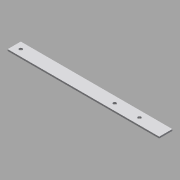
# Autodesk Inventor part: Long Arm
Saved by Autodesk Inventor 2013 (Build 170138000, 138)
## iProperties
Created: 2013-02-08
Part Number: Long Arm
Material: Aluminum 6061-AHC
Document SubType Name: Modeling
Designer: Naphat
Density: 1 g/cm^3
Author: Naphat
Autodesk Inventor part; units mm, degrees
ref_plane "YZ Plane" through (0, 0, 0) normal (1, 0, 0) x (0, 1, 0)
ref_plane "XZ Plane" through (0, 0, 0) normal (0, 1, 0) x (-1, 0, 0)
ref_plane "XY Plane" through (0, 0, 0) normal (0, 0, 1) x (1, 0, 0)
sketch "Sketch1" plane through (0, 0, 0) normal (0, 1, 0) x (-1, 0, 0)
  line L0 (0, 0) -> (0, 25.4)
  line L1 (0, 25.4) -> (254, 25.4)
  line L2 (254, 25.4) -> (254, 0)
  line L3 (254, 0) -> (0, 0)
  dimension "d0" = 25.4
  dimension "d1" = 254
  constraints: 8 end point, 2 perpendicular, 1 parallel, 1 vertical
  measures "d0" distance of L0.start L0.end
  measures "d1" distance of L0.end L1.end
extrude "Extrusion1" add sketch "Sketch1" along normal blind 3
sketch "Sketch2" plane through (0, 3, 0) normal (0, 1, 0) x (1, 0, 0)
  line L0 (0, -25.4) -> (0, 0) projected
  line L1 (0, 0) -> (-254, 0) projected
  line L2 (-254, 0) -> (-254, -25.4) projected
  line L3 (-254, -25.4) -> (0, -25.4) projected
  line L4 (-254, 0) -> (-254, -12.7) construction
  line L5 (-254, 0) -> (-241.3, 0) construction
  line L6 (0, 0) -> (-12.7, 0) construction
  line L7 (0, 0) -> (0, -12.7) construction
  line L8 (0, -12.7) -> (-254, -12.7) construction
  line L9 (-241.3, 0) -> (-241.3, -25.4) construction
  line L10 (-12.7, 0) -> (-12.7, -25.4) construction
  circle A0 centre (-241.3, -12.7) radius 3.175
  circle A1 centre (-12.7, -12.7) radius 3.175
  dimension "d4" = 12.7
  dimension "d5" = 12.7
  dimension "d6" = 12.7
  dimension "d7" = 12.7
  dimension "d8" = 6.35
  dimension "d9" = 6.35
  constraints: 14 end point, 4 midpoint, 4 point on line, 2 centre point, 2 perpendicular
  measures "d4" distance of L1.end L4.end
  measures "d5" distance of L1.end L5.end
  measures "d6" distance of L0.end L6.end
  measures "d7" distance of L0.end L7.end
  measures "d8" diameter of A0
  measures "d9" diameter of A1
hole "Hole1" at (-12.7, 3, 12.7) at (-241.3, 3, 12.7) direction (0, -1, 0) diameter 6.35 depth 25.4 tip angle 118
sketch "Sketch3" plane through (0, 3, 0) normal (0, 1, 0) x (1, 0, 0)
  circle A0 centre (-12.7, -12.7) radius 3.175 projected
  line L0 (-254, -25.4) -> (0, -25.4) projected
  line L1 (-12.7, -12.7) -> (-60.325, -12.7) construction
  circle A1 centre (-60.325, -12.7) radius 3.175
  dimension "d17" = 47.625
  dimension "d18" = 6.35
  constraints: 2 end point, 1 centre point, 1 coincident, 1 parallel
  measures "d17" distance of L1.start L1.end
  measures "d18" diameter of A1
hole "Hole2" at (-60.325, 3, 12.7) direction (0, -1, 0) diameter 6.35 depth 25.4 tip angle 118
sketch "Sketch4" plane through (0, 0, 25.4) normal (1, 0, 0) x (0, 0, -1)
  line L0 (25.4, 0) -> (0, 0) projected
  line L1 (25.4, 0) -> (25.4, 3) projected
  line L2 (0, 3) -> (25.4, 3) projected
  line L3 (0, 0) -> (0, 3) projected
extrude "Extrusion2" add sketch "Sketch4" along normal blind 38.1
equation "\"d4\" = d7"
equation "\"d6\" = d5"
equation "\"d8\" = d9"
body "Solid1"
